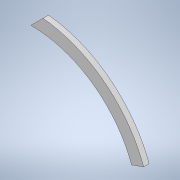
# Autodesk Inventor part: SideA
Saved by Autodesk Inventor 2021.1 (Build 251245010, 245A)
## iProperties
Created: 2020-10-17
Part Number: SideA
Material: Generic
Document SubType Name: Modeling
Designer: robst
Density: 1 g/cm^3
Appearance: Default
Author: robst
Autodesk Inventor part; units mm, degrees
ref_plane "YZ Plane" through (0, 0, 0) normal (1, 0, 0) x (0, 1, 0)
ref_plane "XZ Plane" through (0, 0, 0) normal (0, 1, 0) x (-1, 0, 0)
ref_plane "XY Plane" through (0, 0, 0) normal (0, 0, 1) x (1, 0, 0)
sketch "Sketch1" plane through (0, 0, 0) normal (0, 0, 1) x (1, 0, 0)
  arc A0 (477.3639, 173.7462) -> (8.8135, 507.9235) centre (0, 0) ccw
  arc A1 (469.01, 170.7057) -> (0, 499.11) centre (0, 0) ccw
  arc A2 (525.1002, 191.1209) -> (56.7961, 555.9061) centre (0, 0) ccw
  line L0 (0, 0) -> (0, 499.11)
  line L1 (0, 0) -> (525.1002, 191.1209)
  line L2 (0, 499.11) -> (56.7961, 555.9061)
  dimension "d0" = 1016
  dimension "d1" = 8.89
  dimension "d2" = 50.8
  dimension "d3" = 70
  dimension "d11" = 45
  constraints: 6 end point, 6 point on circle, 3 centre point, 3 coincident, 3 point on line, 1 vertical
  measures "d0" diameter of A0
  measures "d1" radial gap between concentric circles of A1 A0
  measures "d2" radial gap between concentric circles of A2 A0
  measures "d3" angle of L1 L0
  measures "d11" angle of L2 L0
extrude "Extrusion1" add sketch "Sketch1" against normal blind 25.4 contours L1 A1 L2 A0 | A0 L2 A2 L1
sketch "Sketch2" plane through (0, 0, -25.4) normal (0, 0, -1) x (-1, 0, 0)
  circle A0 centre (0, 0) radius 505.46
  circle A1 centre (0, 0) radius 508.635
  arc A2 (0, 499.11) -> (-469.01, 170.7057) centre (0, 0) ccw projected
  dimension "d6" = 3.175
  dimension "d7" = 6.35
  constraints: 2 centre point, 2 coincident
  measures "d6" radial gap between concentric circles of A0 A1
  measures "d7" radial gap between concentric circles of A0 A2
extrude "Extrusion2" cut sketch "Sketch2" against normal blind 19.05
body "Solid1"
